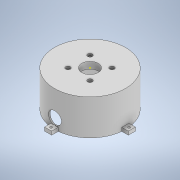
# Autodesk Inventor part: BASE-cilindro
Saved by Autodesk Inventor 2021 (Build 250183000, 183)
## iProperties
Created: 2023-04-04
Part Number: BASE-cilindro
Material: Generic
Document SubType Name: Modeling
Designer: PC
Density: 1 g/cm^3
Appearance: Default
Author: PC
Autodesk Inventor part; units mm, degrees
ref_plane "YZ Plane" through (0, 0, 0) normal (1, 0, 0) x (0, 1, 0)
ref_plane "XY Plane" through (0, 0, 0) normal (0, 0, 1) x (1, 0, 0)
sketch "Sketch1" plane through (0, 0, 0) normal (0, 1, 0) x (-1, 0, 0)
  point P0 (0, 0)
ref_plane "Work Plane26" through (0, 4, 0) normal (0, 1, 0) x (1, 0, 0)
sketch "Sketch2" plane through (0, 4, 0) normal (0, 1, 0) x (1, 0, 0)
  circle A0 centre (0, 0) radius 50
  dimension "d3" = 100
  constraints: 1 centre point, 1 coincident
  measures "d3" diameter of A0
extrude "Base grosor" add sketch "Sketch2" along normal blind 50
ref_plane "Work Plane22" through (0, 54, 0) normal (0, 1, 0) x (1, 0, 0)
sketch "Sketch3" plane through (0, 54, 0) normal (0, 1, 0) x (1, 0, 0)
  circle A0 centre (0, 0) radius 48
  dimension "d6" = 96
  constraints: 1 centre point, 1 coincident
  measures "d6" diameter of A0
extrude "Base agujero" cut sketch "Sketch3" against normal blind 114
sketch "Sketch4" plane through (0, 0, 0) normal (0, 0, 1) x (1, 0, 0)
  circle A0 centre (0, 18.2082) radius 6.6964
  point P0 (0, 0)
  constraints: 1 centre point
extrude "Agujero para cables" cut sketch "Sketch4" along normal blind 89.75
ref_plane "Separacion Tapa" through (0, 54.25, 0) normal (0, 1, 0) x (-1, 0, 0)
ref_plane "Separacion Base Motor" through (0, 36, 0) normal (0, 1, 0) x (1, 0, 0)
sketch "Sketch5" plane through (0, 0, 0) normal (0, 1, 0) x (-1, 0, 0)
  point P0 (0, 0)
sketch "Sketch6" plane through (0, 54.25, 0) normal (0, 1, 0) x (-1, 0, 0)
  point P0 (0, 0)
ref_plane "Work Plane16" through (0, 44.5, 0) normal (0, 1, 0) x (1, 0, 0)
sketch "Sketch127" plane through (0, 44.5, 0) normal (0, 1, 0) x (1, 0, 0)
  circle A0 centre (0, 0) radius 48.8173
  constraints: 1 centre point, 1 coincident
extrude "Extrusion59" add sketch "Sketch127" along normal blind 9.5
ref_plane "Work Plane36" through (0, 54, 0) normal (0, 1, 0) x (1, 0, 0)
sketch "Sketch128" plane through (0, 54, 0) normal (0, 1, 0) x (1, 0, 0)
  circle A0 centre (0, 0) radius 11.5
  line L0 (-15.5, 15.5) -> (15.5, 15.5)
  line L1 (15.5, 15.5) -> (15.5, -15.5)
  line L2 (15.5, -15.5) -> (-15.5, -15.5)
  line L3 (-15.5, -15.5) -> (-15.5, 15.5)
  line L4 (-15.5, 15.5) -> (15.5, -15.5) construction
  line L5 (15.5, 15.5) -> (-15.5, -15.5) construction
  circle A1 centre (-15.5, 15.5) radius 1.55
  circle A2 centre (15.5, 15.5) radius 1.55
  circle A3 centre (15.5, -15.5) radius 1.55
  circle A4 centre (-15.5, -15.5) radius 1.55
  dimension "d231" = 23
  dimension "d232" = 31
  dimension "d233" = 31
  dimension "d234" = 3.1
  dimension "d235" = 3.1
  dimension "d236" = 3.1
  dimension "d237" = 3.1
  constraints: 12 end point, 5 centre point, 4 coincident, 2 midpoint, 2 parallel, 1 horizontal, 1 perpendicular, 1 point on line
  measures "d231" diameter of A0
  measures "d232" distance of L1.end L2.end
  measures "d233" distance of L0.end L1.end
  measures "d234" diameter of A1
  measures "d235" diameter of A2
  measures "d236" diameter of A3
  measures "d237" diameter of A4
extrude "Extrusion60" cut sketch "Sketch128" against normal blind 31 contours A0 | L3 A1 L0 | L0 A1 L3 | A2 L1 L0 | L0 L1 A2 | A4 L2 L3 | L3 L2 A4 | A3 L2 L1 | L1 L2 A3
sketch "Sketch140" plane through (0, 54, 0) normal (0, 1, 0) x (1, 0, 0)
  circle A0 centre (-15.5, 15.5) radius 1.55 projected
  circle A1 centre (-15.5, 15.5) radius 3
  circle A2 centre (15.5, 15.5) radius 1.55 projected
  circle A3 centre (15.5, 15.5) radius 3
  circle A4 centre (-15.5, -15.5) radius 1.55 projected
  circle A5 centre (-15.5, -15.5) radius 3
  circle A6 centre (15.5, -15.5) radius 1.55 projected
  circle A7 centre (15.5, -15.5) radius 3
  point P0 (0, 0)
  dimension "d272" = 6
  dimension "d273" = 6
  dimension "d274" = 6
  dimension "d275" = 6
  constraints: 4 centre point, 4 coincident
  measures "d272" diameter of A1
  measures "d273" diameter of A3
  measures "d274" diameter of A5
  measures "d275" diameter of A7
extrude "Extrusion64" cut sketch "Sketch140" against normal blind 3 contours A0 | A1 | A2 | A3 | A4 | A5 | A6 | A7
ref_plane "Work Plane42" through (0, 0, 44.25) normal (0, 0, 1) x (1, 0, 0)
sketch "Sketch141" plane through (0, 0, 44.25) normal (0, 0, 1) x (1, 0, 0)
  circle A0 centre (0, 17.9692) radius 9
  point P0 (0, 0)
  dimension "d280" = 18
  constraints: 1 centre point
  measures "d280" diameter of A0
extrude "Extrusion65" cut sketch "Sketch141" along normal blind 26.5
sketch "Sketch143" plane through (0, 54, 0) normal (0, 1, 0) x (1, 0, 0)
  circle A0 centre (-15.5, 15.5) radius 1.55 projected
  circle A1 centre (-15.5, 15.5) radius 3.25
  circle A2 centre (15.5, 15.5) radius 1.55 projected
  circle A3 centre (15.5, 15.5) radius 3.25
  circle A4 centre (15.5, -15.5) radius 1.55 projected
  circle A5 centre (15.5, -15.5) radius 3.25
  circle A6 centre (-15.5, -15.5) radius 1.55 projected
  circle A7 centre (-15.5, -15.5) radius 3.25
  point P0 (0, 0)
  dimension "d283" = 6.5
  dimension "d284" = 6.5
  dimension "d285" = 6.5
  dimension "d286" = 6.5
  constraints: 4 centre point, 4 coincident
  measures "d283" diameter of A1
  measures "d284" diameter of A3
  measures "d285" diameter of A5
  measures "d286" diameter of A7
extrude "Extrusion66" cut sketch "Sketch143" against normal blind 3 contours A0 | A1 | A2 | A3 | A4 | A5 | A6 | A7
sketch "Sketch144" plane through (0, 54, 0) normal (0, 1, 0) x (1, 0, 0)
  point P0 (0, 0)
sketch "Sketch145" plane through (0, 0, 0) normal (0, 0, 1) x (1, 0, 0)
  point P0 (0, 0)
sketch "Sketch147" plane through (0, 54, 0) normal (0, 1, 0) x (1, 0, 0)
  point P0 (0, 0)
sketch "Sketch148" plane through (0, 0, 0) normal (0, 1, 0) x (-1, 0, 0)
  point P0 (0, 0)
ref_plane "Work Plane45" through (0, 4, 0) normal (0, 1, 0) x (-1, 0, 0)
sketch "Sketch149" plane through (0, 4, 0) normal (0, 1, 0) x (-1, 0, 0)
  line L0 (-59, -5) -> (-41, -5)
  line L1 (-41, -5) -> (-41, 5)
  line L2 (-41, 5) -> (-59, 5)
  line L3 (-59, 5) -> (-59, -5)
  circle A0 centre (0, 0) radius 50 projected
  line L4 (-59, -5) -> (-41, 5) construction
  line L5 (-41, -5) -> (-59, 5) construction
  line L6 (-49.5364, 8.1105) -> (-49.7724, 8.1105)
  line L7 (-49.7724, 8.1105) -> (-49.7724, 8.4251)
  line L8 (-49.7724, 8.4251) -> (-49.5364, 8.4251)
  line L9 (-49.5364, 8.4251) -> (-49.5364, 8.1105)
  line L10 (-49.5364, 8.1105) -> (-49.7724, 8.4251) construction
  line L11 (-49.7724, 8.1105) -> (-49.5364, 8.4251) construction
  line L12 (-5, 59) -> (5, 59)
  line L13 (5, 59) -> (5, 41)
  line L14 (5, 41) -> (-5, 41)
  line L15 (-5, 41) -> (-5, 59)
  line L16 (-5, 59) -> (5, 41) construction
  line L17 (5, 59) -> (-5, 41) construction
  line L18 (59, 5) -> (41, 5)
  line L19 (41, 5) -> (41, -5)
  line L20 (41, -5) -> (59, -5)
  line L21 (59, -5) -> (59, 5)
  line L22 (59, 5) -> (41, -5) construction
  line L23 (41, 5) -> (59, -5) construction
  line L24 (-5, -41) -> (5, -41)
  line L25 (5, -41) -> (5, -59)
  line L26 (5, -59) -> (-5, -59)
  line L27 (-5, -59) -> (-5, -41)
  line L28 (-5, -41) -> (5, -59) construction
  line L29 (5, -41) -> (-5, -59) construction
  point P0 (-50, 0)
  point P1 (0, 50)
  point P2 (50, 0)
  point P3 (0, -50)
  dimension "d291" = 18
  dimension "d292" = 10
  dimension "d293" = 10
  dimension "d294" = 18
  dimension "d295" = 18
  dimension "d296" = 10
  dimension "d297" = 10
  dimension "d298" = 18
  constraints: 60 end point, 10 parallel, 8 midpoint, 5 horizontal, 5 perpendicular, 4 point on circle
  measures "d291" distance of L2.end L1.end
  measures "d292" distance of L1.end L0.end
  measures "d293" distance of L13.end L14.end
  measures "d294" distance of L12.end L13.end
  measures "d295" distance of L20.end L19.end
  measures "d296" distance of L19.end L18.end
  measures "d297" distance of L25.end L26.end
  measures "d298" distance of L24.end L25.end
extrude "Extrusion67" add sketch "Sketch149" along normal blind 5 contours L3 L2 A0 L0 | A0 L2 L1 L0 | L27 L24 L25 A0 | A0 L25 L26 L27 | L15 L12 L13 A0 | A0 L13 L14 L15 | L20 L19 L18 A0 | A0 L18 L21 L20
sketch "Sketch150" plane through (0, 9, 0) normal (0, 1, 0) x (1, 0, 0)
  circle A0 centre (0, 55.0329) radius 1.55
  circle A1 centre (55.0538, 0) radius 1.55
  circle A2 centre (0, -54.8519) radius 1.55
  circle A3 centre (-54.9513, 0) radius 1.55
  point P0 (0, 0)
  dimension "d301" = 3.1
  dimension "d302" = 3.1
  dimension "d303" = 3.1
  dimension "d304" = 3.1
  constraints: 4 centre point
  measures "d301" diameter of A0
  measures "d302" diameter of A1
  measures "d303" diameter of A2
  measures "d304" diameter of A3
extrude "Extrusion68" cut sketch "Sketch150" against normal blind 12.6
sketch "Sketch151" plane through (0, 9, 0) normal (0, 1, 0) x (1, 0, 0)
  point P0 (0, 0)
sketch "Sketch152" plane through (0, 44.5, 0) normal (0, -1, 0) x (1, 0, 0)
  circle A0 centre (0, 0) radius 48
  constraints: 1 centre point, 1 coincident
extrude "Extrusion69" cut sketch "Sketch152" along normal blind 89.65
sketch "Sketch153" plane through (0, 54, 0) normal (0, 1, 0) x (1, 0, 0)
  point P0 (0, 0)
sketch "Sketch154" plane through (0, 9, 0) normal (0, 1, 0) x (1, 0, 0)
  point P0 (0, 0)
sketch "Sketch155" plane through (0, 54, 0) normal (0, 1, 0) x (1, 0, 0)
  point P0 (0, 0)
sketch "Sketch156" plane through (0, 54, 0) normal (0, 1, 0) x (1, 0, 0)
  point P0 (0, 0)
sketch "Sketch157" plane through (0, 54, 0) normal (0, 1, 0) x (1, 0, 0)
  point P0 (0, 0)
body "Solid1"
